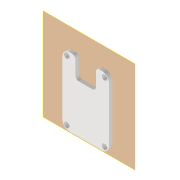
# Autodesk Inventor part: 00_ESP32_XIAO_Adapter_lid
Saved by Autodesk Inventor 2022 (Build 260153000, 153)
## iProperties
Created: 2023-04-27
Part Number: 00_ESP32_XIAO_Adapter_lid
Material: Generisch
Document SubType Name: Modeling
Designer: diederichbenedict
Density: 1 g/cm^3
Appearance: Vorgabe
Author: diederichbenedict
Autodesk Inventor part; units mm, degrees
ref_plane "YZ Plane" through (0, 0, 0) normal (1, 0, 0) x (0, 1, 0)
ref_plane "XZ Plane" through (0, 0, 0) normal (0, 1, 0) x (-1, 0, 0)
ref_plane "XY Plane" through (0, 0, 0) normal (0, 0, 1) x (1, 0, 0)
ref_plane "Arbeitsebene1" through (0, 0, 0) normal (0, 0, 1) x (1, 0, 0)
sketch "Skizze1" plane through (0, 0, 0) normal (0, 0, 1) x (1, 0, 0)
  line L0 (31.9586, -24.4) -> (31.9586, -21.8494) projected
  line L1 (31.9586, -24.4) -> (35.5793, -24.4) projected
  arc A0 (35.5793, -24.4) -> (36.5793, -23.4) centre (35.5793, -23.4) ccw projected
  line L2 (36.5793, -23.4) -> (36.5793, 14.6) projected
  arc A1 (36.5793, 14.6) -> (35.5793, 15.6) centre (35.5793, 14.6) ccw projected
  line L3 (35.5793, 15.6) -> (31.5586, 15.6) projected
  line L4 (31.5586, 15.6) -> (31.5586, -0.3724) projected
  arc A2 (32.766, -2.6793) -> (31.5586, -0.3724) centre (29.9586, -2.6793) ccw projected
  line L5 (32.766, -2.6793) -> (32.766, -19.8793) projected
  arc A3 (31.9586, -21.8494) -> (32.766, -19.8793) centre (29.9586, -19.8793) ccw projected
  line L6 (20.9586, -22.6867) -> (20.9586, -24.4) projected
  line L7 (20.9586, -22.6867) -> (16.1586, -22.6867) projected
  arc A4 (13.3512, -19.8793) -> (16.1586, -22.6867) centre (16.1586, -19.8793) ccw projected
  line L8 (13.3512, -19.8793) -> (13.3512, -2.6793) projected
  arc A5 (14.5586, -0.3724) -> (13.3512, -2.6793) centre (16.1586, -2.6793) ccw projected
  line L9 (14.5586, -0.3724) -> (14.5586, 15.6) projected
  line L10 (14.5586, 15.6) -> (10.5793, 15.6) projected
  arc A6 (10.5793, 15.6) -> (9.5793, 14.6) centre (10.5793, 14.6) ccw projected
  line L11 (9.5793, 14.6) -> (9.5793, -23.4) projected
  arc A7 (9.5793, -23.4) -> (10.5793, -24.4) centre (10.5793, -23.4) ccw projected
  line L12 (10.5793, -24.4) -> (20.9586, -24.4) projected
  circle A8 centre (12.0668, 4.4966) radius 1.4 projected
  line L13 (31.5586, 15.6) -> (14.5586, 15.6)
  line L14 (31.9586, -24.4) -> (20.9586, -24.4)
  line L15 (10.5793, 15.6) -> (9.5793, 15.6)
  line L16 (9.5793, 15.6) -> (9.5793, 14.6)
  line L17 (35.5793, 15.6) -> (36.5793, 15.6)
  line L18 (36.5793, 15.6) -> (36.5793, 14.6)
  line L19 (9.5793, -23.4) -> (9.5793, -24.4)
  line L20 (9.5793, -24.4) -> (10.5793, -24.4)
  line L21 (35.5793, -24.4) -> (36.5793, -24.4)
  line L22 (36.5793, -24.4) -> (36.5793, -23.4)
  constraints: 20 end point, 3 point on line, 2 horizontal, 2 perpendicular, 1 collinear, 1 parallel, 1 vertical
extrude "Extrusion1" add sketch "Skizze1" along normal blind 2 contours L14 L6 L7 A4 L8 A5 L9 L13 L4 A2 L5 A3 L0 | L0 A3 L5 A2 L4 L3 A1 L2 A0 L1 | A0 L22 L21 | L12 A7 L11 A6 L10 L9 A5 L8 A4 L7 L6 | L20 L19 A7 | A1 L17 L18 | L16 L15 A6 | A8
ref_plane "Arbeitsebene2" through (0, 0, 0) normal (0, 0, 1) x (1, 0, 0)
sketch "Skizze2" plane through (0, 0, 2) normal (0, 0, 1) x (1, 0, 0)
  arc A0 (35.5793, -24.4) -> (36.5793, -23.4) centre (35.5793, -23.4) ccw projected
  line L0 (36.5793, -23.4) -> (36.5793, 14.6) projected
  arc A1 (36.5793, 14.6) -> (35.5793, 15.6) centre (35.5793, 14.6) ccw projected
  line L1 (35.5793, 15.6) -> (10.5793, 15.6) projected
  arc A2 (10.5793, 15.6) -> (9.5793, 14.6) centre (10.5793, 14.6) ccw projected
  line L2 (9.5793, 14.6) -> (9.5793, -23.4) projected
  arc A3 (9.5793, -23.4) -> (10.5793, -24.4) centre (10.5793, -23.4) ccw projected
  line L3 (10.5793, -24.4) -> (35.5793, -24.4) projected
  line L4 (34.0793, 13.1) -> (34.0793, -21.9)
  line L5 (34.0793, -21.9) -> (12.0793, -21.9)
  line L6 (12.0793, -21.9) -> (12.0793, 13.1)
  line L7 (12.0793, 13.1) -> (34.0793, 13.1)
  point P0 (8.0712, 15)
  point P1 (8.0712, -15)
  point P2 (38.0712, 15)
  point P3 (38.0712, -15)
  dimension "d21" = 2.5
  constraints: 8 end point, 4 coincident, 3 other
  measures "d21" distance between parallel lines of L0 L4
hole "Bohrung1" at (34.0793, 13.1, 2) at (34.0793, -21.9, 2) at (12.0793, -21.9, 2) at (12.0793, 13.1, 2) direction (0, 0, -1) diameter 3.2 end through all
sketch "Skizze4" plane through (0, 0, 0) normal (0, 0, -1) x (-1, 0, 0)
  circle A0 centre (-34.0793, 13.1) radius 1.4 projected
  circle A1 centre (-34.0793, -21.9) radius 1.4 projected
  line L0 (-31.9586, -24.4) -> (-31.9586, -21.8494) projected
  line L1 (-31.9586, -24.4) -> (-35.5793, -24.4) projected
  arc A2 (-36.5793, -23.4) -> (-35.5793, -24.4) centre (-35.5793, -23.4) ccw projected
  line L2 (-36.5793, -23.4) -> (-36.5793, 14.6) projected
  arc A3 (-35.5793, 15.6) -> (-36.5793, 14.6) centre (-35.5793, 14.6) ccw projected
  line L3 (-35.5793, 15.6) -> (-31.5586, 15.6) projected
  line L4 (-31.5586, 15.6) -> (-31.5586, -0.3724) projected
  arc A4 (-31.5586, -0.3724) -> (-32.766, -2.6793) centre (-29.9586, -2.6793) ccw projected
  line L5 (-32.766, -2.6793) -> (-32.766, -19.8793) projected
  arc A5 (-32.766, -19.8793) -> (-31.9586, -21.8494) centre (-29.9586, -19.8793) ccw projected
  circle A6 centre (-12.0793, -21.9) radius 1.4 projected
  circle A7 centre (-12.0793, 13.1) radius 1.4 projected
  line L6 (-20.9586, -22.6867) -> (-20.9586, -24.4) projected
  line L7 (-20.9586, -22.6867) -> (-16.1586, -22.6867) projected
  arc A8 (-16.1586, -22.6867) -> (-13.3512, -19.8793) centre (-16.1586, -19.8793) ccw projected
  line L8 (-13.3512, -19.8793) -> (-13.3512, -2.6793) projected
  arc A9 (-13.3512, -2.6793) -> (-14.5586, -0.3724) centre (-16.1586, -2.6793) ccw projected
  line L9 (-14.5586, -0.3724) -> (-14.5586, 15.6) projected
  line L10 (-14.5586, 15.6) -> (-10.5793, 15.6) projected
  arc A10 (-9.5793, 14.6) -> (-10.5793, 15.6) centre (-10.5793, 14.6) ccw projected
  line L11 (-9.5793, 14.6) -> (-9.5793, -23.4) projected
  arc A11 (-10.5793, -24.4) -> (-9.5793, -23.4) centre (-10.5793, -23.4) ccw projected
  line L12 (-10.5793, -24.4) -> (-20.9586, -24.4) projected
  circle A12 centre (-12.0668, 4.4966) radius 1.4 projected
  line L13 (-31.0586, -0.651) -> (-31.0586, 16.1)
  line L14 (-31.0586, 16.1) -> (-35.5793, 16.1)
  arc A13 (-35.5793, 16.1) -> (-37.0793, 14.6) centre (-35.5793, 14.6) ccw
  line L15 (-37.0793, 14.6) -> (-37.0793, -23.4)
  arc A14 (-37.0793, -23.4) -> (-35.5793, -24.9) centre (-35.5793, -23.4) ccw
  line L16 (-35.5793, -24.9) -> (-31.4586, -24.9)
  line L17 (-31.4586, -24.9) -> (-31.4586, -21.6326)
  arc A15 (-32.266, -19.8793) -> (-31.4586, -21.6326) centre (-29.9586, -19.8793) ccw
  line L18 (-32.266, -19.8793) -> (-32.266, -2.6793)
  arc A16 (-31.0586, -0.651) -> (-32.266, -2.6793) centre (-29.9586, -2.6793) ccw
  line L19 (-15.0586, 16.1) -> (-15.0586, -0.651)
  arc A17 (-13.8512, -2.6793) -> (-15.0586, -0.651) centre (-16.1586, -2.6793) ccw
  line L20 (-13.8512, -2.6793) -> (-13.8512, -19.8793)
  arc A18 (-16.1586, -22.1867) -> (-13.8512, -19.8793) centre (-16.1586, -19.8793) ccw
  line L21 (-16.1586, -22.1867) -> (-21.4586, -22.1867)
  line L22 (-21.4586, -24.4607) -> (-21.4586, -24.9)
  line L23 (-21.4586, -24.9) -> (-10.5793, -24.9)
  arc A19 (-10.5793, -24.9) -> (-9.0793, -23.4) centre (-10.5793, -23.4) ccw
  line L24 (-9.0793, -23.4) -> (-9.0793, 14.6)
  arc A20 (-9.0793, 14.6) -> (-10.5793, 16.1) centre (-10.5793, 14.6) ccw
  line L25 (-10.5793, 16.1) -> (-15.0586, 16.1)
  line L26 (-31.0586, 15.6607) -> (-15.0586, 15.6607)
  line L27 (-31.4586, -24.4607) -> (-21.4586, -24.4607)
  line L28 (-15.0586, -0.651) -> (-31.0586, -0.651)
  line L29 (-20.9586, -22.6867) -> (-20.9586, -22.1867)
  line L30 (-20.9586, -22.1867) -> (-31.9586, -22.1867)
  point P0 (0, 0)
  point P1 (-31.4586, -22.1867)
  dimension "d22" = 0.5
  dimension "d23" = 0.5
  constraints: 36 end point, 16 point on circle, 8 centre point, 5 point on line, 3 perpendicular, 1 parallel, 17 other
  measures "d22" distance between parallel lines of L4 L13
  measures "d23" distance between parallel lines of L9 L19
extrude "Extrusion2" add sketch "Skizze4" along normal blind 3 contours L17 A15 L18 A16 L28 A17 L20 A18 L21 L30
fillet "Rundung2" radius 4 4 edges at (9.5793, 15.6, 1) (36.5793, 15.6, 1) (9.5793, -24.4, 1) (36.5793, -24.4, 1)
sketch "Skizze5" plane through (0, 0, 0) normal (0, 0, -1) x (-1, 0, 0)
  circle A0 centre (-23.0793, -4.4) radius 4.25 projected
  circle A1 centre (-12.0668, 4.4966) radius 1.4 projected
  circle A2 centre (-34.0668, 4.4966) radius 1.4 projected
  circle A3 centre (-12.0793, 13.1) radius 1.4 projected
  circle A4 centre (-34.0793, -21.9) radius 1.4 projected
  circle A5 centre (-34.0793, 13.1) radius 1.4 projected
  circle A6 centre (-12.0793, -21.9) radius 1.4 projected
  arc A7 (-29.0793, 13.6) -> (-31.0793, 15.6) centre (-31.0793, 13.6) ccw projected
  line L0 (-32.5793, 15.6) -> (-31.0793, 15.6) projected
  arc A8 (-32.5793, 15.6) -> (-36.5793, 11.6) centre (-32.5793, 11.6) ccw projected
  line L1 (-36.5793, -20.4) -> (-36.5793, 11.6) projected
  arc A9 (-36.5793, -20.4) -> (-32.5793, -24.4) centre (-32.5793, -20.4) ccw projected
  line L2 (-13.5793, -24.4) -> (-32.5793, -24.4) projected
  arc A10 (-13.5793, -24.4) -> (-9.5793, -20.4) centre (-13.5793, -20.4) ccw projected
  line L3 (-9.5793, 11.6) -> (-9.5793, -20.4) projected
  arc A11 (-9.5793, 11.6) -> (-13.5793, 15.6) centre (-13.5793, 11.6) ccw projected
  line L4 (-15.0793, 15.6) -> (-13.5793, 15.6) projected
  arc A12 (-15.0793, 15.6) -> (-17.0793, 13.6) centre (-15.0793, 13.6) ccw projected
  line L5 (-17.0793, 13.6) -> (-17.0793, 5.6) projected
  arc A13 (-19.0793, 3.6) -> (-17.0793, 5.6) centre (-19.0793, 5.6) ccw projected
  line L6 (-19.0793, 3.6) -> (-27.0793, 3.6) projected
  arc A14 (-29.0793, 5.6) -> (-27.0793, 3.6) centre (-27.0793, 5.6) ccw projected
  line L7 (-29.0793, 5.6) -> (-29.0793, 13.6) projected
  line L8 (-32.5793, 15.6) -> (-13.5793, 15.6) projected
  point P0 (0, 0)
extrude "Extrusion3" cut sketch "Skizze5" against normal blind 10 contours A7 L8 A12 L5 A13 L6 A14 L7
